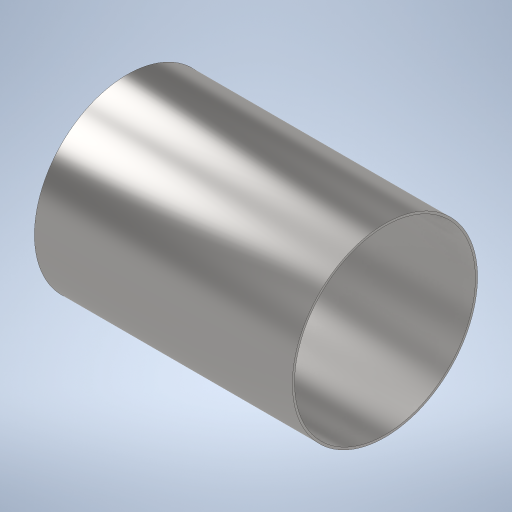
# Autodesk Inventor part: outerwall part 1
Saved by Autodesk Inventor 2023 (Build 270158000, 158)
## iProperties
Created: 2022-07-20
Part Number: outerwall part 1
Material: Stainless Steel
Document SubType Name: Modeling
Designer: station
Density: 8 g/cm^3
Appearance: Semi-Polished
Author: station
Autodesk Inventor part; units mm, degrees
ref_plane "YZ Plane" through (0, 0, 0) normal (1, 0, 0) x (0, 1, 0)
ref_plane "XZ Plane" through (0, 0, 0) normal (0, 1, 0) x (-1, 0, 0)
ref_plane "XY Plane" through (0, 0, 0) normal (0, 0, 1) x (1, 0, 0)
sketch "Sketch1" plane through (0, 0, 0) normal (0, 0, 1) x (1, 0, 0)
  arc A0 (180.1312, 21.4516) -> (182.1847, 21.7676) centre (180.1312, 28.2803) ccw
  arc A1 (166.724, 25.044) -> (180.1312, 21.4516) centre (180.1312, 48.266) ccw
  line L0 (123.3912, 50.0622) -> (166.724, 25.044)
  arc A2 (123.3912, 50.0622) -> (30.0219, 75.0805) centre (30.0219, -111.6581) ccw
  line L1 (0, 75.0805) -> (30.0219, 75.0805)
  line L2 (0, 3.5755) -> (319.1694, 3.5755)
  line L3 (182.1847, 21.7676) -> (237.115, 39.0871)
  line L4 (0, 86.6805) -> (30.0219, 86.6805)
  line L5 (180.1312, 33.0516) -> (237.115, 51.0185)
  line L6 (180.1312, 33.0516) -> (239.8803, 33.0516) construction
  line L7 (0, 88.6805) -> (30.0219, 88.6805)
  line L8 (236.5136, 52.9259) -> (180.1312, 35.1486)
  line L9 (237.115, 51.0185) -> (236.5136, 52.9259)
  line L10 (0, 86.6805) -> (0, 88.6805)
  line L11 (180.1312, 33.0516) -> (180.1312, 35.1486)
  line L12 (180.1312, 33.0516) -> (180.1312, -12.2002)
  line L13 (30.0219, 88.6805) -> (176.1312, 88.6805)
  line L14 (30.0219, 86.6805) -> (178.1312, 86.6805)
  line L15 (176.1312, 88.6805) -> (237.115, 88.6805)
  line L16 (178.1312, 86.6805) -> (237.115, 86.6805)
  line L17 (237.115, 39.0871) -> (237.115, 51.0185)
  line L18 (237.115, 86.6805) -> (237.115, 88.6805)
  point P0 (0, 0)
  dimension "d0" = 30.0219
  dimension "d1" = 186.7386
  dimension "d2" = 0
  dimension "d3" = 0
  dimension "d4" = 71.505
  dimension "d10" = 17.5
  dimension "d11" = 54.9303
  dimension "d13" = 11.6
  dimension "d19" = 17.5
  dimension "d20" = 2
  constraints: 38 end point, 6 point on circle, 5 horizontal, 5 vertical, 3 centre point, 2 parallel, 1 equal length
  measures "d0" distance of L1.start L1.end
  measures "d1" radius of A2
  measures "d2" distance of A2.end L1.end
  measures "d3" distance of L0.start A2.start
  measures "d4" distance between parallel lines of L2 L1
  measures "d10" angle of L2 L3
  measures "d11" horizontal distance of L3.start L3.end
  measures "d13" distance between parallel lines of L1 L4
  measures "d19" angle of L6 L5
  measures "d20" distance between parallel lines of L4 L7
revolve "Revolution4" add sketch "Sketch1" angle 360 about axis through (0, 3.5755, 0) along (1, 0, 0) contours L10 L7 L13 L15 L18 L16 L14 L4
body "Solid4"
